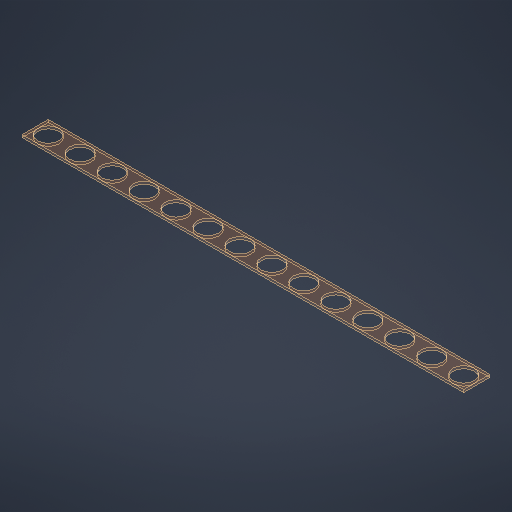
# Autodesk Inventor part: separator-kul
Saved by Autodesk Inventor 2026.1 (Build 301233020, 233B)
## iProperties
Created: 2025-11-04
Part Number: separator-kul
Material: Polycarbonate, Smoke
Document SubType Name: Modeling
Designer: Jan
Density: 1.2 g/cm^3
Appearance: Polycarbonate - Smoked
Author: Jan
Autodesk Inventor part; units mm, degrees
ref_plane "YZ Plane" through (0, 0, 0) normal (1, 0, 0) x (0, 1, 0)
ref_plane "XZ Plane" through (0, 0, 0) normal (0, 1, 0) x (-1, 0, 0)
ref_plane "XY Plane" through (0, 0, 0) normal (0, 0, 1) x (1, 0, 0)
sketch "Sketch1" plane through (0, 0, 0) normal (0, 1, 0) x (-1, 0, 0)
  line L0 (0, 0) -> (-84.3, 0)
  line L1 (-84.3, 0) -> (-84.3, -5)
  line L2 (-84.3, -5) -> (0, -5)
  line L3 (0, -5) -> (0, 0)
  circle A0 centre (-2.5, -2.5) radius 2.05
  circle A1 centre (-8.6, -2.5) radius 2.05
  circle A2 centre (-14.7, -2.5) radius 2.05
  circle A3 centre (-20.8, -2.5) radius 2.05
  circle A4 centre (-26.9, -2.5) radius 2.05
  circle A5 centre (-33, -2.5) radius 2.05
  circle A6 centre (-39.1, -2.5) radius 2.05
  circle A7 centre (-45.2, -2.5) radius 2.05
  circle A8 centre (-51.3, -2.5) radius 2.05
  circle A9 centre (-57.4, -2.5) radius 2.05
  circle A10 centre (-63.5, -2.5) radius 2.05
  circle A11 centre (-69.6, -2.5) radius 2.05
  circle A12 centre (-75.7, -2.5) radius 2.05
  circle A13 centre (-81.8, -2.5) radius 2.05
  dimension "d1" = 5
  dimension "d3" = 4.1
  dimension "d4" = 2.5
  dimension "d5" = 2.5
  dimension "d8" = 6.1
  dimension "d13" = 2.5
  dimension "d16" = 6.1
  dimension "d17" = 4.1
  dimension "d18" = 2.5
  constraints: 14 centre point, 8 end point, 2 horizontal, 2 parallel, 1 coincident, 1 perpendicular, 26 other
  measures "d1" distance of L0.end L1.end
  measures "d3" diameter of A0
  measures "d4" distance from line of L0 A0.centre
  measures "d5" distance from line of L3 A0.centre
  measures "d8" distance of A0.centre A1.centre
  measures "d13" distance from line of A13.centre L1
  measures "d16" distance of A12.centre A13.centre
  measures "d17" diameter of A13
  measures "d18" horizontal distance of A13.centre L0.end
extrude "Extrusion1" add sketch "Sketch1" along normal blind 0.5
equation "\"d5\" = d4"
equation "\"d18\" = d5"
body "Solid1"
